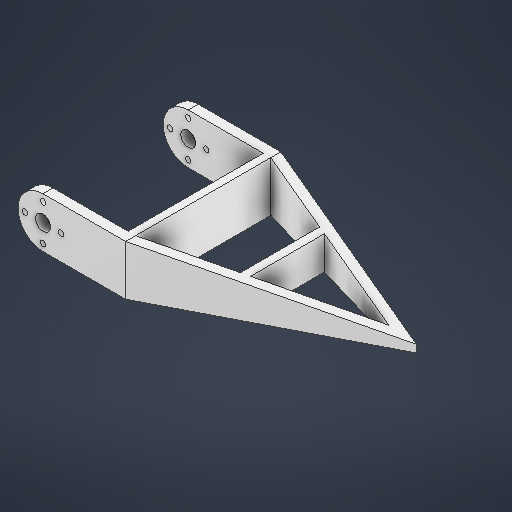
# Autodesk Inventor part: calf_2
Saved by Autodesk Inventor 2026.1 (Build 301233000, 233)
## iProperties
Created: 2025-08-26
Part Number: calf_2
Material: Generic
Document SubType Name: Modeling
Designer: emanuel
Density: 1 g/cm^3
Appearance: Default
Author: emanuel
Autodesk Inventor part; units mm, degrees
ref_plane "YZ Plane" through (0, 0, 0) normal (1, 0, 0) x (0, 1, 0)
ref_plane "XZ Plane" through (0, 0, 0) normal (0, 1, 0) x (-1, 0, 0)
ref_plane "XY Plane" through (0, 0, 0) normal (0, 0, 1) x (1, 0, 0)
sketch "Sketch1" plane through (0, 0, 0) normal (0, 1, 0) x (-1, 0, 0)
  line L0 (0, 0) -> (0, -54)
  line L1 (0, -54) -> (5, -54)
  line L2 (5, -54) -> (5, -58)
  line L3 (5, -58) -> (0, -58)
  line L4 (0, -58) -> (0, -54)
  line L5 (0, 0) -> (3, 0)
  line L6 (3, 0) -> (3, 4)
  line L7 (3, 4) -> (0, 4)
  line L8 (0, 4) -> (0, 0)
  line L9 (3, 0) -> (0, 0)
  line L10 (0, 0) -> (0, -54)
  line L11 (0, -54) -> (3, -54)
  line L12 (3, -54) -> (3, 0)
  line L13 (3, 4) -> (43, 4)
  line L14 (43, 4) -> (43, 0)
  line L15 (43, 0) -> (3, 0)
  line L16 (3, 0) -> (3, 4)
  line L17 (3, -54) -> (43, -54)
  line L18 (43, -54) -> (43, -58)
  line L19 (43, -58) -> (3, -58)
  line L20 (3, -58) -> (3, -54)
  line L21 (0, -27) -> (-82.8143, -27)
  line L22 (-82.8143, -27) -> (-97.578, -27)
  line L23 (0, 4) -> (-84.5723, -26.7818)
  line L24 (0, 4) -> (90, 4) construction
  line L25 (-85.1718, -27) -> (0, -58)
  line L26 (0, 0) -> (-75.1754, -27.3616)
  line L27 (0, 0) -> (80, 0) construction
  line L28 (0, -54) -> (-74.1819, -27)
  line L29 (-32.1773, -27) -> (-32.1773, -42.2884)
  line L30 (-32.1773, -27) -> (-32.1773, -11.7116)
  line L31 (-30.6773, -9.5) -> (-33.6773, -9.5)
  line L32 (-33.6773, -9.5) -> (-33.6773, -44.5)
  line L33 (-33.6773, -44.5) -> (-30.6773, -44.5)
  line L34 (-30.6773, -44.5) -> (-30.6773, -9.5)
  line L35 (-30.6773, -9.5) -> (-33.6773, -44.5) construction
  line L36 (-33.6773, -9.5) -> (-30.6773, -44.5) construction
  line L37 (-84.5723, -26.7818) -> (-85.1718, -27)
  point P0 (-30.6773, -11.1656)
  point P1 (-30.6773, -42.8344)
  point P2 (3, 0)
  point P3 (-33.6773, -41.7424)
  point P4 (-33.6773, -12.2576)
  dimension "d0" = 54
  dimension "d1" = 5
  dimension "d2" = 4
  dimension "d3" = 3
  dimension "d4" = 4
  dimension "d5" = 40
  dimension "d6" = 40
  dimension "d7" = 90
  dimension "d8" = 160
  dimension "d9" = 80
  dimension "d10" = 160
  dimension "d11" = 3
  dimension "d12" = 35
  constraints: 76 end point, 12 parallel, 10 horizontal, 10 point on line, 7 perpendicular, 3 midpoint, 2 equal length, 1 vertical
  measures "d0" distance of L0.start L0.end
  measures "d1" distance of L2.end L3.end
  measures "d2" distance of L1.end L2.end
  measures "d3" distance of L7.end L6.end
  measures "d4" distance of L6.end L5.end
  measures "d5" distance of L14.end L15.end
  measures "d6" distance of L18.end L19.end
  measures "d7" distance of L7.end L23.end
  measures "d8" angle of L23 L24
  measures "d9" distance of L9.end L26.end
  measures "d10" angle of L26 L27
  measures "d11" distance of L33.end L32.end
  measures "d12" distance of L32.end L31.end
extrude "Extrusion1" add sketch "Sketch1" along normal blind 20 contours L5 L12 L1 L0 | L8 L7 L6 L5 | L26 L34 L31 L32 L21 L22 L37 L23 L8 | L6 L13 L14 L15 | L34 L21 L30 L26 | L26 L32 L31 L34 | L1 L20 L3 L4 | L4 L25 L22 L21 L28 L32 L33 L34 | L34 L28 L29 L21 | L1 L2 L3 L20 | L30 L21 L32 L26 | L34 L33 L32 L28 | L29 L28 L32 L21 | L17 L18 L19 L2
sketch "Sketch2" plane through (-43, 0, 4) normal (0, 0, 1) x (1, 0, 0)
  line L0 (43, 20) -> (0, 20) projected
  line L1 (0, 20) -> (10, 20)
  line L2 (10, 20) -> (10, 10)
  line L3 (10, 10) -> (0, 10)
  line L4 (0, 10) -> (0, 20)
  circle A0 centre (10, 10) radius 3
  circle A1 centre (10, 10) radius 10
  line L5 (128.1718, 0) -> (128.1718, 20) projected
  line L6 (128.1718, 10) -> (128.1718, 11.5)
  line L7 (128.1718, 11.5) -> (128.1718, 8.5)
  line L8 (43, 0) -> (0, 0) projected
  line L9 (128.1718, 8.5) -> (43, 0)
  line L10 (43, 0) -> (128.1718, 0)
  line L11 (128.1718, 0) -> (128.1718, 8.5)
  line L12 (43, 20) -> (73.6773, 20) projected
  line L13 (128.1718, 11.5) -> (43, 20)
  line L14 (128.1718, 20) -> (43, 20) projected
  line L15 (43, 20) -> (128.1718, 20)
  line L16 (128.1718, 20) -> (128.1718, 11.5)
  line L17 (10, 10) -> (0, 10)
  line L18 (0, 10) -> (0, 0)
  line L19 (0, 0) -> (10, 0)
  line L20 (10, 0) -> (10, 10)
  circle A2 centre (10, 10) radius 8
  circle A3 centre (10, 10) radius 6.5
  line L21 (10, 18) -> (10, 16.5)
  circle A4 centre (10, 17.25) radius 1.1
  line L22 (2, 10) -> (3.5, 10)
  circle A5 centre (2.75, 10) radius 1.1
  line L23 (10, 3.5) -> (10, 2)
  circle A6 centre (10, 2.75) radius 1.1
  line L24 (16.5, 10) -> (18, 10)
  circle A7 centre (17.25, 10) radius 1.1
  dimension "d15" = 10
  dimension "d16" = 10
  dimension "d17" = 6
  dimension "d18" = 1.5
  dimension "d19" = 3
  dimension "d22" = 16
  dimension "d23" = 13
  dimension "d24" = 2.2
  dimension "d25" = 2.2
  dimension "d26" = 2.2
  dimension "d27" = 2.2
  constraints: 40 end point, 8 point on circle, 8 point on line, 7 centre point, 5 midpoint, 5 parallel, 4 coincident, 4 perpendicular, 3 horizontal, 1 collinear, 1 vertical, 3 other
  measures "d15" distance of L2.end L3.end
  measures "d16" distance of L1.end L2.end
  measures "d17" diameter of A0
  measures "d18" distance of L6.start L6.end
  measures "d19" distance of L6.end L7.end
  measures "d22" diameter of A2
  measures "d23" diameter of A3
  measures "d24" diameter of A4
  measures "d25" diameter of A5
  measures "d26" diameter of A6
  measures "d27" diameter of A7
extrude "Extrusion2" cut sketch "Sketch2" against normal blind 100 contours L12 L14 L5 L13 | A1 L4 L0 | A4 A2 L2 | L2 A2 A4 | A1 L8 L18 | A2 A4 A3 L2 | L2 A3 A4 A2 | A5 A2 L3 | L3 A2 A5 | L5 L10 L9 | A3 A4 L2 | L2 A4 A3 | A7 A2 | A2 L24 A3 A7 | A5 A3 L3 A2 | A6 A2 L20 | L20 A2 A6 | L3 A3 A5 A2 | A2 A7 A3 L24 | A3 A7 | A5 L3 A3 | A2 A6 A3 L20 | L20 A3 A6 A2 | L3 A5 A3 | A0 L20 L2 | L2 L3 A0 | A3 A6 L20 | L20 A6 A3 | L20 A0 L3
body "Solid1"
